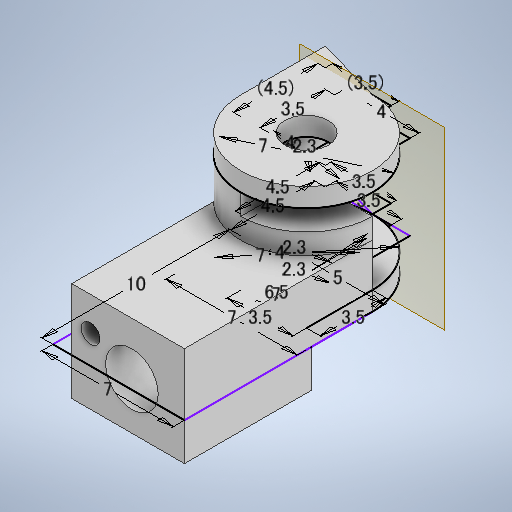
# Autodesk Inventor part: trod2.0
Saved by Autodesk Inventor 2025 (Build 290162000, 162)
## iProperties
Created: 2024-07-30
Part Number: trod2.0
Material: 一般
Document SubType Name: Modeling
Designer: Saigusa
Density: 1 g/cm^3
Appearance: 既定
Author: Saigusa
Autodesk Inventor part; units mm, degrees
ref_plane "YZ Plane" through (0, 0, 0) normal (1, 0, 0) x (0, 1, 0)
ref_plane "XZ Plane" through (0, 0, 0) normal (0, 1, 0) x (-1, 0, 0)
ref_plane "XY Plane" through (0, 0, 0) normal (0, 0, 1) x (1, 0, 0)
sketch "スケッチ1" plane through (0, 0, 0) normal (0, 1, 0) x (-1, 0, 0)
  circle A0 centre (0, 0) radius 1.15
  circle A1 centre (0, 0) radius 2
  circle A2 centre (0, 0) radius 3.5
  line L0 (0, 0) -> (-3.5, 0)
  line L1 (-3.5, 0) -> (-3.5, 3.5)
  line L2 (-3.5, 3.5) -> (0, 3.5)
  line L3 (0, 3.5) -> (0, 0)
  line L4 (-2, 0) -> (2, 0)
  line L5 (2, 0) -> (2, -3.5)
  line L6 (2, -3.5) -> (-2, -3.5)
  line L7 (-2, -3.5) -> (-2, 0)
  line L8 (0, 0) -> (3.5, 0)
  line L9 (3.5, 0) -> (3.5, -4.5)
  line L10 (3.5, -4.5) -> (0, -4.5)
  line L11 (0, -4.5) -> (0, 0)
  line L12 (0, -3.5) -> (3.5, -4.5)
  line L13 (2, -3.5) -> (2, -4.5)
  point P0 (0, 2)
  point P1 (2, -2.8723)
  point P2 (2, -4.0714)
  dimension "d1" = 4
  dimension "d0" = 2.3
  dimension "d2" = 7
  dimension "d3" = 3.5
  dimension "d4" = 3.5
  dimension "d41" = 3.5
  dimension "d42" = 4.5
  constraints: 28 end point, 6 parallel, 4 perpendicular, 3 coincident, 3 horizontal, 3 point on line, 2 centre point, 1 midpoint, 3 other
  measures "d0" diameter of A0
  measures "d2" diameter of A2
  measures "d3" distance of L1.end L2.end
  measures "d4" distance of L0.end L1.end
  measures "d41" distance of L9.end L10.end
  measures "d42" distance of L8.end L9.end
extrude "押し出し1" add sketch "スケッチ1" along normal blind 3.4 contours A1 L0 A2 L3
extrude "押し出し2" add sketch "スケッチ1" along normal blind 4.5 contours L8 A2 L5 | A1 L3 A2 L8 | A2 L9 L12 L13 L5
extrude "押し出し3" add sketch "スケッチ1" against normal blind 1 contours L4 A1 L11 A0 | A0 L3 A1 L4 | A0 L0 A1 L3 | L11 A1 L0 A0 | L5 A2 L11 A1 | L8 A2 L5 | A1 L3 A2 L8 | A1 L0 A2 L3 | L11 A2 L7 A1 | L7 A2 L0
sketch "スケッチ2" plane through (0, 4.5, 0) normal (0, 1, 0) x (1, 0, 0)
  circle A0 centre (0, 0) radius 1.15
  circle A1 centre (0, 0) radius 2
  circle A2 centre (0, 0) radius 3.5
  line L0 (2, 0) -> (-2, 0)
  line L1 (-2, 0) -> (-2, 3.5)
  line L2 (-2, 3.5) -> (2, 3.5)
  line L3 (2, 3.5) -> (2, 0)
  line L4 (-3.5, 4.5) -> (-3.5, 0) projected
  line L5 (0, 0) -> (-3.5, 0)
  line L6 (-3.5, 0) -> (-3.5, 4.5)
  line L7 (-3.5, 4.5) -> (0, 4.5)
  line L8 (0, 4.5) -> (0, 0)
  line L9 (0, 3.5) -> (-3.5, 4.5)
  line L10 (-2, 2.8723) -> (-2, 4.0714) projected
  line L11 (-2, 0) -> (-2, 4.0714)
  point P0 (0, 3.5)
  dimension "d12" = 4
  dimension "d11" = 2.3
  dimension "d13" = 7
  dimension "d14" = 4
  dimension "d15" = 3.5
  dimension "d43" = 3.5
  dimension "d44" = 4.5
  constraints: 20 end point, 4 parallel, 3 coincident, 2 centre point, 2 horizontal, 2 perpendicular, 1 collinear, 1 horizontal alignment, 1 midpoint, 1 point on line, 2 other
  measures "d11" diameter of A0
  measures "d13" diameter of A2
  measures "d14" distance of L1.end L2.end
  measures "d15" distance of L0.end L1.end
  measures "d43" distance of L4.start L7.end
  measures "d44" distance of L5.end L4.start
extrude "押し出し4" add sketch "スケッチ2" along normal blind 1 contours L0 A1 A0 | A0 L8 A1 L0 | A0 L0 A1 L8 | L3 A2 L5 A1 | A1 L8 A2 L3 | A1 L1 A2 L8 | L5 A2 L1 | A2 L1 L2 | L2 L10 L9 | A2 L4 L9 L10 L1
sketch "スケッチ3" plane through (0, -1, 0) normal (0, -1, 0) x (1, 0, 0)
  circle A0 centre (0, 0) radius 1.15
  circle A1 centre (0, 0) radius 3.5
  line L0 (-3.5, 0) -> (3.5, 0)
  line L1 (3.5, 0) -> (3.5, 3.5)
  line L2 (3.5, 3.5) -> (-3.5, 3.5)
  line L3 (-3.5, 3.5) -> (-3.5, 0)
  line L4 (0, 0) -> (3.5, 0)
  line L5 (3.5, 0) -> (3.5, 3.5)
  line L6 (3.5, 3.5) -> (0, 3.5)
  line L7 (0, 3.5) -> (0, 0)
  line L8 (3.5, 0) -> (-3.5, 0)
  line L9 (-3.5, 0) -> (-3.5, 10)
  line L10 (-3.5, 10) -> (3.5, 10)
  line L11 (3.5, 10) -> (3.5, 0)
  line L12 (3.5, 10) -> (-1.5, 10)
  line L13 (-1.5, 10) -> (-1.5, 0)
  line L14 (-1.5, 0) -> (3.5, 0)
  line L15 (3.5, 0) -> (3.5, 10)
  line L16 (-3.5, 0) -> (-1.5, 0)
  line L17 (-1.5, 0) -> (-2.5, 0)
  line L18 (-2.5, 0) -> (-2.5, 10)
  circle A2 centre (0, 0) radius 3.25
  line L19 (0, 3.25) -> (3.5, 3.25)
  line L20 (3.5, 3.25) -> (3.5, 3.5)
  line L21 (3.5, 3.5) -> (0, 3.5)
  line L22 (0, 3.5) -> (0, 3.25)
  line L23 (0, 0) -> (-3.5, 0)
  line L24 (-3.5, 0) -> (-3.5, -4.5)
  line L25 (-3.5, -4.5) -> (0, -4.5)
  line L26 (0, -4.5) -> (0, 0)
  line L27 (0, -3.5) -> (-3.5, -4.5)
  point P0 (0, 3.5)
  point P1 (-1.5, 3.1623)
  point P2 (-2.5, 2.4495)
  point P3 (-2.5, 2.0767)
  dimension "d33" = 6.5
  dimension "d18" = 2.3
  dimension "d19" = 7
  dimension "d20" = 7
  dimension "d23" = 7
  dimension "d24" = 10
  dimension "d25" = 5
  dimension "d39" = 3.5
  dimension "d40" = 4.5
  constraints: 56 end point, 12 parallel, 7 perpendicular, 6 horizontal, 4 point on line, 3 coincident, 2 centre point, 2 point on circle, 1 collinear, 1 midpoint, 3 other
  measures "d18" diameter of A0
  measures "d19" diameter of A1
  measures "d20" distance of L2.end L1.end
  measures "d23" distance of L9.end L10.end
  measures "d24" distance of L8.end L9.end
  measures "d25" distance of L14.end L13.end
  measures "d39" distance of L25.end L24.end
  measures "d40" distance of L24.end L23.end
extrude "押し出し5" add sketch "スケッチ3" against normal blind 3.3 contours A1 L19 L1 | L2 L1 L19 A1 | L2 L13 L10 L11 | A1 L13 L2 | A1 L18 L2 L13 | L2 L18 L10 L13
extrude "押し出し6" add sketch "スケッチ3" along normal blind 2 contours A2 L13 A1 L7 | L7 A1 L19 | L2 L1 L19 A1 | L2 L13 L10 L11 | A1 L13 L2 | A2 L18 A1 L13 | A1 L18 L2 L13 | L2 L18 L10 L13
ref_plane "作業平面1" through (-2, 0, -3.5) normal (0, 0, 1) x (1, 0, 0)
sketch "スケッチ4" plane through (-2, 0, -3.5) normal (0, 0, 1) x (1, 0, 0)
  line L0 (2, 3.4) -> (2, 0)
  line L1 (2, 0) -> (2, 0.5)
  line L2 (2, 0.5) -> (0.5, 0.5)
  circle A0 centre (0.5, 0.5) radius 0.5
  line L3 (0, 0) -> (4, 0) projected
  dimension "d28" = 0.5
  dimension "d29" = 1.5
  dimension "d30" = 90
  constraints: 6 end point, 1 centre point, 1 coincident, 1 perpendicular, 1 point on line, 1 tangent, 1 vertical
  measures "d28" distance of L0.end L1.end
  measures "d29" distance of L1.end L2.end
  measures "d30" angle of L2 L1
extrude "押し出し7" cut sketch "スケッチ4" along normal blind 20 contours A0
sketch "スケッチ5" plane through (-2.5, 2.3, 10) normal (0, 0, 1) x (1, 0, 0)
  line L0 (6, -3.3) -> (6, -5.3) projected
  line L1 (6, -5.3) -> (3.2, -5.3)
  line L2 (3.2, -5.3) -> (3.2, -2.8)
  line L3 (3.2, -2.8) -> (6, -2.8)
  line L4 (6, -2.8) -> (6, -5.3)
  circle A0 centre (3.2, -2.8) radius 1.4
  point P0 (2.5, -2.3)
  dimension "d34" = 2.8
  dimension "d35" = 2.5
  dimension "d36" = 2.8
  constraints: 8 end point, 2 parallel, 1 centre point, 1 coincident, 1 horizontal, 1 perpendicular
  measures "d34" distance of L2.end L3.end
  measures "d35" distance of L1.end L2.end
  measures "d36" diameter of A0
extrude "押し出し8" cut sketch "スケッチ5" against normal blind 5 contours A0 L2 L3 | L3 L2 A0
extrude "押し出し9" add sketch "スケッチ3" against normal blind 1 contours L27 L24 A1
